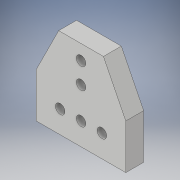
# Autodesk Inventor part: nhk47
Saved by Autodesk Inventor 2019 (Build 230136000, 136)
## iProperties
Created: 2022-02-27
Part Number: nhk47
Material: 一般
Document SubType Name: Sheet Metal
Designer: yuta
Density: 1 g/cm^3
Sheet Metal Rule: Default_mm
Appearance: 既定
Author: yuta
Autodesk Inventor part; units mm, degrees
ref_plane "YZ Plane" through (0, 0, 0) normal (1, 0, 0) x (0, 1, 0)
ref_plane "XZ Plane" through (0, 0, 0) normal (0, 1, 0) x (-1, 0, 0)
ref_plane "XY Plane" through (0, 0, 0) normal (0, 0, 1) x (1, 0, 0)
sketch "スケッチ1" plane through (0, 0, 0) normal (0, 0, 1) x (1, 0, 0)
  line L0 (0, 0) -> (30, 0)
  line L1 (30, 0) -> (30, 15)
  line L2 (22.5, 30) -> (7.5, 30)
  line L3 (0, 15) -> (0, 0)
  line L4 (0, 15) -> (7.5, 30)
  line L5 (22.5, 30) -> (30, 15)
  dimension "d2" = 15
  dimension "d5" = 15
  dimension "d6" = 15
  dimension "d7" = 26.565
  dimension "d8" = 26.565
  constraints: 12 end point, 2 parallel, 1 horizontal, 1 perpendicular
  measures "d2" distance of L3.start L0.start
  measures "d5" distance of L2.end L2.start
  measures "d6" distance from line of L1.end L0
  measures "d7" angle of L1 L5
  measures "d8" angle of L3 L4
extrude "押し出し1" add sketch "スケッチ1" along normal blind 6
sketch "スケッチ2" plane through (0, 0, 6) normal (0, 0, 1) x (1, 0, 0)
  circle A0 centre (15, 7.5) radius 1.6
  line L0 (0, 0) -> (30, 0) projected
  line L1 (0, 15) -> (0, 0) projected
  circle A1 centre (8, 7.5) radius 1.6
  circle A2 centre (22, 7.5) radius 1.6
  circle A3 centre (15, 25) radius 1.6
  line L2 (22.5, 30) -> (7.5, 30) projected
  circle A4 centre (15, 18) radius 1.6
  dimension "d11" = 3.2
  dimension "d12" = 7.5
  dimension "d13" = 15
  dimension "d14" = 3.2
  dimension "d15" = 3.2
  dimension "d16" = 7
  dimension "d17" = 7
  dimension "d18" = 3.2
  dimension "d19" = 5
  dimension "d20" = 3.2
  dimension "d21" = 7
  constraints: 5 centre point
  measures "d11" diameter of A0
  measures "d12" distance from line of L0 A0.centre
  measures "d13" distance from line of L1 A0.centre
  measures "d14" diameter of A1
  measures "d15" diameter of A2
  measures "d16" distance of A0.centre A1.centre
  measures "d17" distance of A2.centre A0.centre
  measures "d18" diameter of A3
  measures "d19" distance from line of A3.centre L2
  measures "d20" diameter of A4
  measures "d21" distance of A3.centre A4.centre
hole "穴1" at (15, 18, 6) at (15, 25, 6) at (8, 7.5, 6) at (15, 7.5, 6) at (22, 7.5, 6) direction (0, 0, -1) diameter 3.2 depth 6
equation "\"BendRadius\" = Thickness"
equation "\"BendReliefWidth\" = Thickness"
equation "\"BendReliefDepth\" = 0.5 * Thickness"
equation "\"CornerReliefSize\" = 4 * Thickness"
equation "\"MinimumRemnant\" = 2 * Thickness"
equation "\"TransitionRadius\" = BendRadius"
equation "\"JacobiRadiusSize\" = BendRadius"
equation "\"GapSize\" = Thickness"
equation "\"Thickness\" = 0.5"
